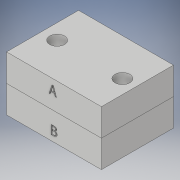
# Autodesk Inventor part: 5_8-Cap
Saved by Autodesk Inventor 2019.3 (Build 233278000, 278)
## iProperties
Created: 2018-12-29
Part Number: 5_8-Cap
Material: Generic
Document SubType Name: Modeling
Designer: eroldan
Density: 1 g/cm^3
Appearance: Default
Author: eroldan
Autodesk Inventor part; units mm, degrees
ref_plane "YZ Plane" through (0, 0, 0) normal (1, 0, 0) x (0, 1, 0)
ref_plane "XZ Plane" through (0, 0, 0) normal (0, 1, 0) x (-1, 0, 0)
ref_plane "XY Plane" through (0, 0, 0) normal (0, 0, 1) x (1, 0, 0)
sketch "Sketch1" plane through (0, 0, 0) normal (0, 0, 1) x (1, 0, 0)
  circle A0 centre (0, 0) radius 7.9375
  circle A1 centre (0, 0) radius 7
  dimension "d0" = 15.875
  dimension "d1" = 14
  constraints: 2 centre point, 2 coincident
  measures "d0" diameter of A0
  measures "d1" diameter of A1
extrude "Extrusion1" add sketch "Sketch1" against normal blind 3
extrude "Extrusion2" add sketch "Sketch1" against normal blind 17.75 contours A1
sketch "Sketch2" plane through (0, 0, 0) normal (0, 1, 0) x (-1, 0, 0)
  line L0 (7, -4.1691) -> (5, -5.8103)
  line L1 (5, -5.8103) -> (7, -5.8103)
  line L2 (0, -24) -> (0, 4) projected
  line L3 (7, -3) -> (7, -17.75) projected
  point P0 (0, 0)
  dimension "d9" = 2
  constraints: 4 end point, 2 point on line, 1 perpendicular
  measures "d9" distance of L0.end L1.end
revolve "Revolution2" cut sketch "Sketch2" angle 360 about axis through (0, 0, -10) along (0, 0, 1)
fillet "Fillet1" radius 0.5 1 edges at (5, 0, -5.8103)
pattern_linear "Rectangular Pattern1" count 3 spacing 4 along (0, 0, -1) of "Revolution2", "Fillet1"
fillet "Fillet2" radius 2 2 edges at (-7.9375, 0, 0) (-7, 0, -17.75)
sketch "Sketch3" plane through (0, 0, 0) normal (0, 1, 0) x (-1, 0, 0)
  line L0 (16.2755, -22.2142) -> (-16.3359, -22.2142)
  line L1 (-16.3359, -22.2142) -> (-16.3359, 2.5379)
  line L2 (-16.3359, 2.5379) -> (16.2755, 2.5379)
  line L3 (16.2755, 2.5379) -> (16.2755, -22.2142)
  point P0 (0, 0)
  constraints: 8 end point, 2 parallel, 1 horizontal, 1 perpendicular
extrude "Extrusion3" add sketch "Sketch3" along normal mid plane 18.75 separate body
sketch "Sketch6" plane through (-16.2755, 9.375, 2.5379) normal (0, 0, 1) x (1, 0, 0)
  line L0 (14.6317, -1.9631) -> (19.2729, -1.9631) construction
  line L1 (19.2729, -1.9631) -> (19.2729, -5.0111) construction
  line L2 (19.2729, -5.0111) -> (14.6317, -5.0111) construction
  line L3 (14.6317, -5.0111) -> (14.6317, -1.9631) construction
  line L4 (15.0208, -13.9038) -> (17.4909, -13.9038) construction
  line L5 (17.4909, -13.9038) -> (17.4909, -16.9518) construction
  line L6 (17.4909, -16.9518) -> (15.0208, -16.9518) construction
  line L7 (15.0208, -16.9518) -> (15.0208, -13.9038) construction
  line L8 (14.6119, -5.0111) -> (15.6395, -1.9631)
  line L9 (15.6395, -1.9631) -> (16.1384, -1.9631)
  line L10 (16.1384, -1.9631) -> (17.1659, -5.0111)
  line L11 (17.1659, -5.0111) -> (16.7386, -5.0111)
  line L12 (16.7386, -5.0111) -> (16.462, -4.159)
  line L13 (16.462, -4.159) -> (15.2986, -4.159)
  line L14 (15.2986, -4.159) -> (15.022, -5.0111)
  line L15 (15.022, -5.0111) -> (14.6119, -5.0111)
  line L16 (16.3508, -3.8131) -> (15.8791, -2.3781)
  line L17 (15.8791, -2.3781) -> (15.4098, -3.8131)
  line L18 (15.4098, -3.8131) -> (16.3508, -3.8131)
  spline S0 degree 2 poles (17.397, -16.0157) (17.397, -16.2429) (17.2241, -16.5912) (17.0808, -16.7048) knots 0 0 0 1 2 2 2
  spline S1 degree 2 poles (17.0808, -16.7048) (16.9079, -16.8382) (16.5152, -16.9518) (16.204, -16.9518) knots 0 0 0 1 2 2 2
  line L19 (16.204, -16.9518) -> (15.3296, -16.9518)
  line L20 (15.3296, -16.9518) -> (15.3296, -13.9038)
  line L21 (15.3296, -13.9038) -> (16.1373, -13.9038)
  spline S2 degree 2 poles (16.1373, -13.9038) (16.4633, -13.9038) (16.7894, -13.9458) (16.9376, -14.0273) knots 0 0 0 1 2 2 2
  spline S3 degree 2 poles (16.9376, -14.0273) (17.1031, -14.1137) (17.2537, -14.3978) (17.2537, -14.5905) knots 0 0 0 1 2 2 2
  spline S4 degree 2 poles (17.2537, -14.5905) (17.2537, -14.8054) (17.0265, -15.1462) (16.8264, -15.2425) knots 0 0 0 1 2 2 2
  line L22 (16.8264, -15.2425) -> (16.8264, -15.2574)
  spline S5 degree 2 poles (16.8264, -15.2574) (17.0981, -15.3315) (17.397, -15.7242) (17.397, -16.0157) knots 0 0 0 1 2 2 2
  spline S6 degree 2 poles (16.9746, -16.0329) (16.9746, -15.86) (16.8758, -15.6377) (16.7276, -15.5587) knots 0 0 0 1 2 2 2
  spline S7 degree 2 poles (16.7276, -15.5587) (16.6313, -15.5093) (16.4041, -15.4797) (16.1941, -15.4797) knots 0 0 0 1 2 2 2
  line L23 (16.1941, -15.4797) -> (15.7347, -15.4797)
  line L24 (15.7347, -15.4797) -> (15.7347, -16.606)
  line L25 (15.7347, -16.606) -> (16.0632, -16.606)
  spline S8 degree 2 poles (16.0632, -16.606) (16.33, -16.606) (16.6362, -16.5566) (16.7548, -16.4776) knots 0 0 0 1 2 2 2
  spline S9 degree 2 poles (16.7548, -16.4776) (16.8684, -16.396) (16.9746, -16.1935) (16.9746, -16.0329) knots 0 0 0 1 2 2 2
  spline S10 degree 2 poles (16.8314, -14.6473) (16.8314, -14.5386) (16.7573, -14.3756) (16.6758, -14.3286) knots 0 0 0 1 2 2 2
  spline S11 degree 2 poles (16.6758, -14.3286) (16.577, -14.2743) (16.3374, -14.2496) (16.1225, -14.2496) knots 0 0 0 1 2 2 2
  line L26 (16.1225, -14.2496) -> (15.7347, -14.2496)
  line L27 (15.7347, -14.2496) -> (15.7347, -15.1413)
  line L28 (15.7347, -15.1413) -> (16.1941, -15.1413)
  spline S12 degree 2 poles (16.1941, -15.1413) (16.3843, -15.1413) (16.5646, -15.1018) (16.6609, -15.04) knots 0 0 0 1 2 2 2
  spline S13 degree 2 poles (16.6609, -15.04) (16.7548, -14.9807) (16.8314, -14.7905) (16.8314, -14.6473) knots 0 0 0 1 2 2 2
  point P0 (16.2755, -9.375)
  constraints: 4 other
emboss "Emboss1" sketch "Sketch6" operation cut depth 0.5 direction (0, 0, -1)
sketch "Sketch4" plane through (0, 9.375, 0) normal (0, 1, 0) x (1, 0, 0)
  point P0 (0, 0)
  point P1 (11.5671, 9.4399)
  point P2 (-11.0549, 9.6289)
hole "Hole1" at (11.5671, 9.375, -9.4399) at (-11.0549, 9.375, -9.6289) direction (0, -1, 0) diameter 5.1 end through all both bodies 2
combine bodies "Combine1" operation type subtract main body 2 bodies to subtract 1
split body "Split1" result two bodies by plane through (0, 0, 0) normal (0, 1, 0) bodies 2 first body at (-3.1012, 8.875, -18.6553)
